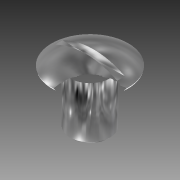
# Autodesk Inventor part: screw
Saved by Autodesk Inventor 2014 (Build 180170000, 170)
## iProperties
Shininess: 86.0
Length Units: 11272
Angle Units: 11279
Time Units: 11290
Mass Units: 11286
Length Display Precision: 3
Angle Display Precision: 2
Compacted: True
Created: 2001-07-10
Part Number: screw
Document SubType Name: Modeling
Designer: Autodesk, Inc.
Mass: 0.168196 g
Surface Area: 0.603871 cm^2
Volume: 0.0208164 cm^3
Density: 8.08 g/cm^3
Material: Stainless Steel
Appearance: Chrome - Polished
Density: 0.0
Volumn: 0.0
Area: 0.0
PropertySet Name: Model Information
Control State: 0
Master: False
Checked Out: False
Author: Autodesk, Inc.
Autodesk Inventor part; units mm, degrees
ref_plane "YZ Plane" through (0, 0, 0) normal (1, 0, 0) x (0, 1, 0)
ref_plane "XZ Plane" through (0, 0, 0) normal (0, 1, 0) x (-1, 0, 0)
ref_plane "XY Plane" through (0, 0, 0) normal (0, 0, 1) x (1, 0, 0)
sketch "Sketch1" plane through (0, 0, 0) normal (0, 0, 1) x (1, 0, 0)
  line L0 (0, 3.9687) -> (0, 0)
  line L1 (0, 0) -> (1.1906, 0)
  line L2 (1.1906, 0) -> (1.1906, 3.175)
  line L3 (1.1906, 3.175) -> (2.3813, 3.175)
  arc A0 (2.3813, 3.175) -> (0, 3.9687) centre (0, 0) ccw
  line L4 (0, 3.9687) -> (11.1125, 3.9688)
  dimension "d1" = 1.1906
  dimension "d2" = 2.3813
  dimension "d3" = 0.7937
  constraints: 10 end point, 2 parallel, 2 point on circle, 1 centre point, 1 perpendicular, 1 tangent, 1 vertical
  measures "d1" distance of L2.end L3.end
  measures "d2" distance from line of L3.end L0
  measures "d3" distance between parallel lines of L4 L3
revolve "Revolution1" add sketch "Sketch1" angle 360 about axis through (0, 3.9687, 0) along (0, -1, 0)
chamfer "Chamfer1" distance 0.127 angle 45 2 edges at (-1.1906, 0, 0) (-2.3813, 3.175, 0)
sketch "Sketch2" plane through (0, 0, 0) normal (1, 0, 0) x (0, 1, 0)
  line L0 (3.5066, 0.2385) -> (4.5681, 0.2385)
  line L1 (4.5681, 0.2385) -> (4.5681, -0.2201)
  line L2 (4.5681, -0.2201) -> (3.5066, -0.2201)
  line L3 (3.5066, -0.2201) -> (3.5066, 0.2385)
  constraints: 8 end point, 2 parallel, 1 horizontal, 1 perpendicular
extrude "Extrusion1" cut sketch "Sketch2" against normal mid plane 25.4
equation "\"d1\" = 0.5 * d2"
body "Solid1"
